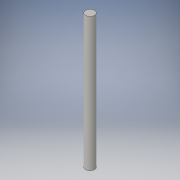
# Autodesk Inventor part: pitchingMachineThrowerAxel
Saved by Autodesk Inventor 2016 SP1 (Build 200210100, 210)
## iProperties
Created: 2016-01-12
Part Number: pitchingMachineThrowerAxel
Material: Generic
Document SubType Name: Modeling
Designer: steele
Density: 1 g/cm^3
Appearance: Default
Author: steele
Autodesk Inventor part; units mm, degrees
ref_plane "YZ Plane" through (0, 0, 0) normal (1, 0, 0) x (0, 1, 0)
ref_plane "XZ Plane" through (0, 0, 0) normal (0, 1, 0) x (-1, 0, 0)
ref_plane "XY Plane" through (0, 0, 0) normal (0, 0, 1) x (1, 0, 0)
sketch "Sketch2" plane through (0, 0, 0) normal (0, 1, 0) x (-1, 0, 0)
  circle A0 centre (0, 0) radius 5.08
  dimension "d0" = 10.16
  constraints: 1 centre point, 1 coincident
  measures "d0" diameter of A0
extrude "Extrusion1" add sketch "Sketch2" along normal mid plane 152.4
equation "\"d0\" = pMThrowerHubDiam"
equation "\"d1\" = pmThrowererHubLength"
equation "\"pMThrowerHubDiam\" = 10.16"
equation "\"pmThrowererHubLength\" = 152.4"
body "Solid1"
